Autodesk Fusion 360 part; units mm, degrees
note: some values were not read from the file. Chosen so that the rebuilt part matches the saved one: which bodies a step acts on. Set by a fixed rule: which sketch regions a step uses.
(part 2 of 3)
sketch "Esquisse32" plane through (0, 0, -500) normal (0, 0, -1) x (-1, 0, 0)
  line L0 (-249.6527, -49.4848) -> (-249.7286, -49.4459)
  spline S0 degree 5 poles (-249.7286, -49.4459) (-249.7324, -49.3927) (-249.7363, -49.3397) (-249.7403, -49.2867) (-249.7444, -49.2339) (-249.7485, -49.1812) knots 0.023756 0.023756 0.023756 0.023756 0.023756 0.023756 0.032153 0.032153 0.032153 0.032153 0.032153 0.032153
  spline S1 degree 5 poles (-249.7485, -49.1812) (-249.7705, -49.2534) (-249.7926, -49.3259) (-249.8149, -49.3986) (-249.8372, -49.4715) (-249.8597, -49.5447) knots 0.980595 0.980595 0.980595 0.980595 0.980595 0.980595 0.989283 0.989283 0.989283 0.989283 0.989283 0.989283
  line L1 (-249.8597, -49.5447) -> (-249.8814, -49.5038)
  line L2 (-249.8814, -49.5038) -> (-249.8118, -49.3682)
  spline S2 degree 5 poles (-249.8118, -49.3682) (-249.8339, -49.38) (-249.8559, -49.3918) (-249.878, -49.4036) (-249.9, -49.4154) (-249.922, -49.4272) knots 0 0 0 0 0 0 0.003856 0.003856 0.003856 0.003856 0.003856 0.003856
  spline S3 degree 5 poles (-249.922, -49.4272) (-249.9554, -49.364) (-249.989, -49.3006) (-250.0226, -49.237) (-250.0563, -49.1731) (-250.0901, -49.109) knots 0.991923 0.991923 0.991923 0.991923 0.991923 0.991923 1 1 1 1 1 1
  spline S4 degree 5 poles (-250.0901, -49.109) (-250.1008, -49.1968) (-250.1112, -49.2844) (-250.1213, -49.3717) (-250.1312, -49.4588) (-250.1409, -49.5456) knots 0 0 0 0 0 0 0.013626 0.013626 0.013626 0.013626 0.013626 0.013626
  line L3 (-250.1409, -49.5456) -> (-250.1797, -49.5667)
  spline S5 degree 5 poles (-250.1797, -49.5667) (-251.1535, -48.3219) (-253.072, -45.9257) (-255.5912, -42.9683) (-258.2607, -40.2233) (-260.8003, -38.1712) (-262.454, -37.2128) (-263.5373, -36.7637) (-264.1941, -36.5764) (-264.5063, -36.5108) knots -0.98163 -0.98163 -0.98163 -0.98163 -0.98163 -0.98163 -0.8 -0.6 -0.4 -0.2 0 0 0 0 0 0
  spline S6 degree 5 poles (-264.5063, -36.5108) (-263.9407, -36.3998) (-262.8337, -36.2121) (-261.2449, -36.0334) (-259.2727, -36.0041) (-257.0669, -36.3389) (-255.1423, -37.076) (-253.5194, -38.2446) (-252.2045, -39.8541) (-251.1806, -41.88) (-250.4724, -44.1331) (-250.0804, -46.1405) (-249.8774, -47.72) (-249.7819, -48.7553) (-249.7485, -49.1812) knots -1 -1 -1 -1 -1 -1 -0.9 -0.8 -0.7 -0.6 -0.5 -0.4 -0.3 -0.2 -0.1 -0.032153 -0.032153 -0.032153 -0.032153 -0.032153 -0.032153
  spline S7 degree 5 poles (-249.7485, -49.1812) (-249.2912, -47.6805) (-248.4329, -44.7466) (-247.4586, -40.9967) (-246.7428, -37.2421) (-246.5187, -33.9882) (-246.6822, -32.0838) (-246.9356, -30.9388) (-247.159, -30.2933) (-247.2842, -30) knots -0.980595 -0.980595 -0.980595 -0.980595 -0.980595 -0.980595 -0.8 -0.6 -0.4 -0.2 0 0 0 0 0 0
  spline S8 degree 5 poles (-247.2842, -30) (-246.8689, -30.3996) (-246.0802, -31.1988) (-245.0225, -32.3977) (-243.8673, -33.9965) (-242.8764, -35.9953) (-242.3763, -37.9947) (-242.4027, -39.9944) (-242.9669, -41.9947) (-244.0392, -43.9954) (-245.4301, -45.8049) (-246.7771, -47.2143) (-247.8695, -48.2236) (-248.5742, -48.8326) (-248.821, -49.0413) knots -1 -1 -1 -1 -1 -1 -0.9 -0.8 -0.7 -0.6 -0.5 -0.4 -0.3 -0.2 -0.1 -0.047889 -0.047889 -0.047889 -0.047889 -0.047889 -0.047889
  spline S9 degree 5 poles (-248.821, -49.0413) (-247.5601, -48.3647) (-245.0121, -46.9618) (-241.7841, -45.0562) (-238.692, -42.9485) (-236.2638, -40.8331) (-235.0328, -39.3709) (-234.4024, -38.3821) (-234.1038, -37.7677) (-233.985, -37.4718) knots -0.968205 -0.968205 -0.968205 -0.968205 -0.968205 -0.968205 -0.8 -0.6 -0.4 -0.2 0 0 0 0 0 0
  spline S10 degree 5 poles (-233.985, -37.4718) (-233.9739, -38.0479) (-233.9813, -39.1708) (-234.0812, -40.7664) (-234.3948, -42.7138) (-235.1075, -44.8279) (-236.1676, -46.5953) (-237.6004, -47.9907) (-239.4137, -49.0061) (-241.5866, -49.6626) (-243.9284, -49.9689) (-245.9734, -50.0063) (-247.5642, -49.9319) (-248.6004, -49.8462) (-249.0256, -49.8051) knots -1 -1 -1 -1 -1 -1 -0.9 -0.8 -0.7 -0.6 -0.5 -0.4 -0.3 -0.2 -0.1 -0.032153 -0.032153 -0.032153 -0.032153 -0.032153 -0.032153
  spline S11 degree 5 poles (-249.0256, -49.8051) (-247.6271, -50.5161) (-244.8868, -51.8708) (-241.3631, -53.4815) (-237.7898, -54.8384) (-234.6242, -55.6241) (-232.7204, -55.7938) (-231.5488, -55.743) (-230.8743, -55.6352) (-230.5637, -55.5627) knots -0.980595 -0.980595 -0.980595 -0.980595 -0.980595 -0.980595 -0.8 -0.6 -0.4 -0.2 0 0 0 0 0 0
  spline S12 degree 5 poles (-230.5637, -55.5627) (-231.0293, -55.9023) (-231.9534, -56.5403) (-233.3177, -57.3737) (-235.0928, -58.2338) (-237.2334, -58.8625) (-239.2892, -59.0079) (-241.254, -58.6346) (-243.1259, -57.7316) (-244.91, -56.3282) (-246.5742, -54.509) (-247.8421, -52.746) (-248.755, -51.2735) (-249.3394, -50.243) (-249.6109, -49.7443) knots -1 -1 -1 -1 -1 -1 -0.9 -0.8 -0.7 -0.6 -0.5 -0.4 -0.3 -0.2 -0.1 -0.011578 -0.011578 -0.011578 -0.011578 -0.011578 -0.011578
  spline S13 degree 5 poles (-249.6109, -49.7443) (-249.4929, -49.7574) (-249.3754, -49.7701) (-249.2583, -49.7822) (-249.1417, -49.7939) (-249.0256, -49.8051) knots 0.013626 0.013626 0.013626 0.013626 0.013626 0.013626 0.032153 0.032153 0.032153 0.032153 0.032153 0.032153
  spline S14 degree 5 poles (-249.0256, -49.8051) (-249.1138, -49.7603) (-249.2023, -49.7152) (-249.2913, -49.6698) (-249.3806, -49.6242) (-249.4703, -49.5783) knots 0.980595 0.980595 0.980595 0.980595 0.980595 0.980595 0.99198 0.99198 0.99198 0.99198 0.99198 0.99198
  spline S15 degree 5 poles (-249.4703, -49.5783) (-249.3376, -49.4709) (-249.2064, -49.3635) (-249.0765, -49.2561) (-248.9481, -49.1487) (-248.821, -49.0413) knots 0.021065 0.021065 0.021065 0.021065 0.021065 0.021065 0.047889 0.047889 0.047889 0.047889 0.047889 0.047889
  spline S16 degree 5 poles (-248.821, -49.0413) (-248.9841, -49.1288) (-249.1488, -49.2169) (-249.3152, -49.3056) (-249.4831, -49.3949) (-249.6527, -49.4848) knots 0.968205 0.968205 0.968205 0.968205 0.968205 0.968205 0.989961 0.989961 0.989961 0.989961 0.989961 0.989961
  line L4 (-250.1023, -49.9358) -> (-250.0313, -49.9578)
  spline S17 degree 5 poles (-250.0313, -49.9578) (-250.0413, -49.9451) (-250.0513, -49.9323) (-250.0612, -49.9197) (-250.0712, -49.907) (-250.0812, -49.8943) knots 0 0 0 0 0 0 0.002489 0.002489 0.002489 0.002489 0.002489 0.002489
  line L5 (-250.0812, -49.8943) -> (-250.0337, -49.8013)
  line L6 (-250.0337, -49.8013) -> (-250.0105, -49.7833)
  line L7 (-250.0105, -49.7833) -> (-249.955, -49.8544)
  line L8 (-249.955, -49.8544) -> (-250, -50)
  spline S18 degree 5 poles (-250, -50) (-249.9803, -49.9846) (-249.9606, -49.9691) (-249.941, -49.9537) (-249.9213, -49.9382) (-249.9018, -49.9228) knots 0 0 0 0 0 0 0.003856 0.003856 0.003856 0.003856 0.003856 0.003856
  spline S19 degree 5 poles (-249.9018, -49.9228) (-249.8578, -49.9792) (-249.8138, -50.0358) (-249.7696, -50.0927) (-249.7253, -50.1497) (-249.6809, -50.207) knots 0.991923 0.991923 0.991923 0.991923 0.991923 0.991923 1 1 1 1 1 1
  spline S20 degree 5 poles (-249.6809, -50.207) (-249.6849, -50.1334) (-249.689, -50.06) (-249.6932, -49.9868) (-249.6976, -49.9138) (-249.7021, -49.8411) knots 0 0 0 0 0 0 0.01135 0.01135 0.01135 0.01135 0.01135 0.01135
  spline S21 degree 5 poles (-249.7021, -49.8411) (-248.9612, -51.2322) (-247.49, -53.9208) (-245.5244, -57.2671) (-243.3735, -60.4318) (-241.2297, -62.8927) (-239.7674, -64.1237) (-238.7786, -64.7541) (-238.1643, -65.0527) (-237.8683, -65.1715) knots -0.98124 -0.98124 -0.98124 -0.98124 -0.98124 -0.98124 -0.8 -0.6 -0.4 -0.2 0 0 0 0 0 0
  spline S22 degree 5 poles (-237.8683, -65.1715) (-238.4445, -65.1826) (-239.5673, -65.1752) (-241.163, -65.0753) (-243.1104, -64.7617) (-245.2245, -64.049) (-246.9918, -62.9889) (-248.3872, -61.5561) (-249.4026, -59.7428) (-250.0592, -57.5699) (-250.3654, -55.2281) (-250.4028, -53.1831) (-250.3285, -51.5923) (-250.2427, -50.5561) (-250.2017, -50.1309) knots -1 -1 -1 -1 -1 -1 -0.9 -0.8 -0.7 -0.6 -0.5 -0.4 -0.3 -0.2 -0.1 -0.032153 -0.032153 -0.032153 -0.032153 -0.032153 -0.032153
  spline S23 degree 5 poles (-250.2017, -50.1309) (-250.9126, -51.5294) (-252.2674, -54.2697) (-253.878, -57.7934) (-255.2349, -61.3667) (-256.0206, -64.5323) (-256.1903, -66.4361) (-256.1395, -67.6077) (-256.0317, -68.2822) (-255.9593, -68.5928) knots -0.980595 -0.980595 -0.980595 -0.980595 -0.980595 -0.980595 -0.8 -0.6 -0.4 -0.2 0 0 0 0 0 0
  spline S24 degree 5 poles (-255.9593, -68.5928) (-256.2989, -68.1272) (-256.9369, -67.2031) (-257.7703, -65.8388) (-258.6303, -64.0637) (-259.2591, -61.9231) (-259.3879, -60.1012) (-259.1823, -58.744) (-258.8808, -57.8097) (-258.6501, -57.269) (-258.5758, -57.1069) knots -1 -1 -1 -1 -1 -1 -0.9 -0.8 -0.7 -0.6 -0.5 -0.456879 -0.456879 -0.456879 -0.456879 -0.456879 -0.456879
  spline S25 degree 5 poles (-258.5758, -57.1069) (-258.7531, -57.2839) (-259.561, -58.1021) (-260.775, -59.4308) (-262.0352, -61.0602) (-262.8185, -62.4118) (-263.2676, -63.4951) (-263.4549, -64.1519) (-263.5206, -64.464) knots -0.653826 -0.653826 -0.653826 -0.653826 -0.653826 -0.653826 -0.6 -0.4 -0.2 0 0 0 0 0 0
  spline S26 degree 5 poles (-263.5206, -64.464) (-263.6315, -63.8985) (-263.8192, -62.7915) (-263.998, -61.2027) (-264.0273, -59.2305) (-263.6925, -57.0247) (-262.9554, -55.1001) (-261.7867, -53.4771) (-260.1772, -52.1622) (-258.1513, -51.1384) (-255.8983, -50.4301) (-253.8908, -50.0382) (-252.3113, -49.8352) (-251.276, -49.7397) (-250.8501, -49.7063) knots -1 -1 -1 -1 -1 -1 -0.9 -0.8 -0.7 -0.6 -0.5 -0.4 -0.3 -0.2 -0.1 -0.032153 -0.032153 -0.032153 -0.032153 -0.032153 -0.032153
  spline S27 degree 5 poles (-250.8501, -49.7063) (-252.3508, -49.2489) (-255.2848, -48.3906) (-259.0346, -47.4164) (-262.7892, -46.7005) (-266.029, -46.4775) (-267.9273, -46.6383) (-269.0681, -46.888) (-269.7105, -47.1073) (-270, -47.2287) knots -0.980595 -0.980595 -0.980595 -0.980595 -0.980595 -0.980595 -0.8 -0.6 -0.4 -0.2 -0.004255 -0.004255 -0.004255 -0.004255 -0.004255 -0.004255
  line L9 (-270, -47.2287) -> (-270, -47.2095)
  spline S28 degree 5 poles (-270, -47.2095) (-269.6067, -46.802) (-268.8137, -46.0214) (-267.6211, -44.9712) (-266.0286, -43.822) (-264.036, -42.8342) (-262.0367, -42.334) (-260.0369, -42.3604) (-258.0366, -42.9247) (-256.0359, -43.9969) (-254.0869, -45.4951) (-252.5378, -47.0043) (-251.3889, -48.2878) (-250.6403, -49.1926) (-250.292, -49.6283) knots -0.998432 -0.998432 -0.998432 -0.998432 -0.998432 -0.998432 -0.9 -0.8 -0.7 -0.6 -0.5 -0.4 -0.3 -0.2 -0.1 -0.013022 -0.013022 -0.013022 -0.013022 -0.013022 -0.013022
  spline S29 degree 5 poles (-250.292, -49.6283) (-250.3077, -49.6369) (-250.3234, -49.6456) (-250.3391, -49.6542) (-250.3548, -49.6629) (-250.3704, -49.6715) knots 0.016959 0.016959 0.016959 0.016959 0.016959 0.016959 0.019765 0.019765 0.019765 0.019765 0.019765 0.019765
  spline S30 degree 5 poles (-250.3704, -49.6715) (-250.4671, -49.678) (-250.5634, -49.6846) (-250.6593, -49.6916) (-250.7549, -49.6988) (-250.8501, -49.7063) knots 0.016987 0.016987 0.016987 0.016987 0.016987 0.016987 0.032153 0.032153 0.032153 0.032153 0.032153 0.032153
  spline S31 degree 5 poles (-250.8501, -49.7063) (-250.7965, -49.7226) (-250.7428, -49.739) (-250.6889, -49.7555) (-250.6349, -49.772) (-250.5808, -49.7886) knots 0.980595 0.980595 0.980595 0.980595 0.980595 0.980595 0.987045 0.987045 0.987045 0.987045 0.987045 0.987045
  spline S32 degree 5 poles (-250.5808, -49.7886) (-250.9817, -50.0133) (-251.9101, -50.5515) (-253.2852, -51.4174) (-254.9643, -52.6361) (-256.5642, -54.0996) (-257.6012, -55.3668) (-258.1844, -56.3076) (-258.4778, -56.8931) (-258.5758, -57.1069) knots 0.027348 0.027348 0.027348 0.027348 0.027348 0.027348 0.1 0.2 0.3 0.4 0.456879 0.456879 0.456879 0.456879 0.456879 0.456879
  spline S33 degree 5 poles (-258.5758, -57.1069) (-258.0942, -56.6262) (-256.885, -55.4616) (-255.4179, -54.1468) (-253.6373, -52.6494) (-251.5014, -50.945) (-250.1803, -49.9154) knots 0.653826 0.653826 0.653826 0.653826 0.653826 0.653826 0.8 0.989864 0.989864 0.989864 0.989864 0.989864 0.989864
  spline S34 degree 5 poles (-250.1803, -49.9154) (-250.1847, -49.9586) (-250.189, -50.0018) (-250.1933, -50.0449) (-250.1975, -50.0879) (-250.2017, -50.1309) knots 0.025297 0.025297 0.025297 0.025297 0.025297 0.025297 0.032153 0.032153 0.032153 0.032153 0.032153 0.032153
  spline S35 degree 5 poles (-250.2017, -50.1309) (-250.1819, -50.092) (-250.1621, -50.0531) (-250.1422, -50.0141) (-250.1223, -49.975) (-250.1023, -49.9358) knots 0.980595 0.980595 0.980595 0.980595 0.980595 0.980595 0.985614 0.985614 0.985614 0.985614 0.985614 0.985614
  line L10 (0, 0) -> (-500, 0)
  line L11 (-500, 0) -> (-500, -100)
  line L12 (-500, -100) -> (0, -100)
  line L13 (0, -100) -> (0, 0)
  spline S36 degree 5 poles (-752.6094, 2.3587) (-751.4125, 3.3722) (-749.2008, 5.4108) (-746.6033, 8.4178) (-744.8759, 12.1299) (-745.0448, 16.2519) (-746.2254, 20.0781) (-746.9511, 23.8392) (-746.165, 27.5533) (-743.8381, 30.7762) (-740.6502, 32.8311) (-737.642, 33.0469) (-735.8698, 31.0183) (-736.1134, 26.7853) (-738.8366, 20.7166) (-744.0362, 13.4698) (-751.253, 5.8891) (-759.2111, -0.975) (-766.2809, -6.1031) (-768.9611, -8.1361) (-765.9148, -6.7187) (-760.6181, -3.5743) (-756.3821, -0.6706) (-753.8063, 1.3451) (-752.6094, 2.3587) knots 0 0 0 0 0 0 0.05 0.1 0.15 0.2 0.25 0.3 0.35 0.4 0.45 0.5 0.55 0.6 0.65 0.7 0.75 0.8 0.85 0.9 0.95 1 1 1 1 1 1
  line L14 (-761.998, -2.9349) -> (-767.7728, -7.266)
  spline S37 degree 5 poles (-752.6094, 2.3587) (-752.294, 3.293) (-751.7934, 5.1547) (-751.451, 7.8793) (-751.7283, 11.3123) (-752.6342, 15.4745) (-753.2774, 19.8274) (-752.9808, 24.5534) (-751.5025, 29.4566) (-749.3688, 33.6811) (-747.5009, 36.1011) (-746.8345, 35.7156) (-747.8954, 32.0962) (-750.5345, 25.6604) (-754.1877, 17.3561) (-758.0383, 8.4584) (-761.2107, 0.3317) (-762.9503, -5.7913) (-762.8064, -9.035) (-760.8298, -9.1227) (-757.7438, -6.5899) (-755.2007, -3.2383) (-753.6859, -0.4512) (-752.9248, 1.4243) (-752.6094, 2.3587) knots 0 0 0 0 0 0 0.05 0.1 0.15 0.2 0.25 0.3 0.35 0.4 0.45 0.5 0.55 0.6 0.65 0.7 0.75 0.8 0.85 0.9 0.95 1 1 1 1 1 1
  spline S38 degree 5 poles (-752.6094, 2.3587) (-752.5578, 3.3434) (-752.5781, 5.2711) (-752.9834, 7.9872) (-754.1766, 11.218) (-756.1719, 14.9814) (-757.9657, 18.9993) (-758.9551, 23.6302) (-758.8544, 28.7504) (-757.9396, 33.3939) (-756.794, 36.2281) (-756.0482, 36.0366) (-756.0933, 32.2653) (-756.8982, 25.3561) (-758.1755, 16.3741) (-759.4827, 6.7675) (-760.3449, -1.9137) (-760.368, -8.279) (-759.3543, -11.3636) (-757.4273, -10.9148) (-755.1392, -7.6433) (-753.5946, -3.7299) (-752.8879, -0.6375) (-752.661, 1.3739) (-752.6094, 2.3587) knots 0 0 0 0 0 0 0.05 0.1 0.15 0.2 0.25 0.3 0.35 0.4 0.45 0.5 0.55 0.6 0.65 0.7 0.75 0.8 0.85 0.9 0.95 1 1 1 1 1 1
  spline S39 degree 5 poles (-752.6094, 2.3587) (-752.8254, 3.3208) (-753.365, 5.1716) (-754.4881, 7.6775) (-756.5087, 10.4667) (-759.4454, 13.5522) (-762.2566, 16.9371) (-764.4588, 21.1293) (-765.7433, 26.0868) (-766.1152, 30.8049) (-765.7767, 33.8431) (-765.0069, 33.86) (-764.0328, 30.2163) (-762.9438, 23.3462) (-761.7504, 14.3527) (-760.4173, 4.7496) (-758.9054, -3.8423) (-757.2103, -9.9778) (-755.4019, -12.6745) (-753.6675, -11.7224) (-752.3469, -7.9549) (-751.9154, -3.7699) (-752.0692, -0.6015) (-752.3934, 1.3965) (-752.6094, 2.3587) knots 0 0 0 0 0 0 0.05 0.1 0.15 0.2 0.25 0.3 0.35 0.4 0.45 0.5 0.55 0.6 0.65 0.7 0.75 0.8 0.85 0.9 0.95 1 1 1 1 1 1
  spline S40 degree 5 poles (-752.6094, 2.3587) (-753.0769, 3.2269) (-754.0959, 4.8634) (-755.8534, 6.9734) (-758.5517, 9.114) (-762.2118, 11.2928) (-765.8321, 13.7937) (-769.0836, 17.2363) (-771.658, 21.6634) (-773.289, 26.1062) (-773.7828, 29.1231) (-773.0461, 29.347) (-771.1251, 26.1012) (-768.2229, 19.7797) (-764.6474, 11.4417) (-760.7728, 2.5544) (-756.9989, -5.311) (-753.7114, -10.7617) (-751.2425, -12.8705) (-749.8293, -11.4857) (-749.574, -7.5016) (-750.2876, -3.3554) (-751.2906, -0.346) (-752.1418, 1.4904) (-752.6094, 2.3587) knots 0 0 0 0 0 0 0.05 0.1 0.15 0.2 0.25 0.3 0.35 0.4 0.45 0.5 0.55 0.6 0.65 0.7 0.75 0.8 0.85 0.9 0.95 1 1 1 1 1 1
  spline S41 degree 5 poles (-752.6094, 2.3587) (-753.2938, 3.0685) (-754.7165, 4.3695) (-756.9782, 5.9271) (-760.1539, 7.2603) (-764.2662, 8.3708) (-768.4269, 9.8022) (-772.4867, 12.2399) (-776.16, 15.8083) (-778.9292, 19.6463) (-780.2186, 22.4181) (-779.5697, 22.8325) (-776.8442, 20.2253) (-772.3441, 14.9212) (-766.6515, 7.8571) (-760.5229, 0.3447) (-754.7669, -6.2109) (-750.1307, -10.5724) (-747.1844, -11.9369) (-746.1972, -10.2223) (-747.0263, -6.317) (-748.8321, -2.5171) (-750.6098, 0.1101) (-751.9249, 1.6488) (-752.6094, 2.3587) knots 0 0 0 0 0 0 0.05 0.1 0.15 0.2 0.25 0.3 0.35 0.4 0.45 0.5 0.55 0.6 0.65 0.7 0.75 0.8 0.85 0.9 0.95 1 1 1 1 1 1
  spline S42 degree 5 poles (-752.6094, 2.3587) (-753.46, 2.8576) (-755.1809, 3.7264) (-757.7789, 4.6161) (-761.1965, 5.043) (-765.456, 5.0029) (-769.8486, 5.2587) (-774.4155, 6.5107) (-778.9153, 8.9557) (-782.6174, 11.9042) (-784.6068, 14.2254) (-784.0937, 14.7994) (-780.7658, 13.0243) (-775.0016, 9.131) (-767.6143, 3.8647) (-759.6861, -1.7157) (-752.3748, -6.4752) (-746.7338, -9.4242) (-743.5287, -9.9432) (-743.0407, -8.0257) (-744.8927, -4.489) (-747.6567, -1.3172) (-750.0773, 0.733) (-751.7588, 1.8598) (-752.6094, 2.3587) knots 0 0 0 0 0 0 0.05 0.1 0.15 0.2 0.25 0.3 0.35 0.4 0.45 0.5 0.55 0.6 0.65 0.7 0.75 0.8 0.85 0.9 0.95 1 1 1 1 1 1
  spline S43 degree 5 poles (-752.6094, 2.3587) (-753.5631, 2.6096) (-755.4546, 2.9819) (-758.1963, 3.1376) (-761.6023, 2.6267) (-765.693, 1.4389) (-769.9918, 0.5001) (-774.7271, 0.4735) (-779.7197, 1.6138) (-784.0799, 3.4542) (-786.6218, 5.1525) (-786.2826, 5.8438) (-782.5993, 5.0323) (-775.9984, 2.8385) (-767.4642, -0.2395) (-758.3244, -3.4739) (-750.0002, -6.0843) (-743.7728, -7.402) (-740.5464, -7.037) (-740.5938, -5.0591) (-743.3313, -2.1532) (-746.8486, 0.1553) (-749.7326, 1.4764) (-751.6557, 2.1077) (-752.6094, 2.3587) knots 0 0 0 0 0 0 0.05 0.1 0.15 0.2 0.25 0.3 0.35 0.4 0.45 0.5 0.55 0.6 0.65 0.7 0.75 0.8 0.85 0.9 0.95 1 1 1 1 1 1
  spline S44 degree 5 poles (-752.6094, 2.3587) (-753.5954, 2.343) (-755.5172, 2.1912) (-758.1993, 1.6014) (-761.3412, 0.1905) (-764.9596, -2.0569) (-768.8458, -4.1207) (-773.3983, -5.4239) (-778.5134, -5.6729) (-783.2085, -5.0771) (-786.1143, -4.1275) (-785.9742, -3.3704) (-782.2085, -3.158) (-775.2605, -3.4896) (-766.2123, -4.1509) (-756.5389, -4.7995) (-747.8191, -5.0673) (-741.467, -4.656) (-738.4588, -3.4341) (-739.0381, -1.5422) (-742.4581, 0.5173) (-746.4678, 1.7913) (-749.6013, 2.2853) (-751.6234, 2.3743) (-752.6094, 2.3587) knots 0 0 0 0 0 0 0.05 0.1 0.15 0.2 0.25 0.3 0.35 0.4 0.45 0.5 0.55 0.6 0.65 0.7 0.75 0.8 0.85 0.9 0.95 1 1 1 1 1 1
  spline S45 degree 5 poles (-752.6094, 2.3587) (-753.5546, 2.0775) (-755.3642, 1.4129) (-757.7877, 0.1214) (-760.4324, -2.0849) (-763.3104, -5.2252) (-766.4955, -8.261) (-770.5276, -10.7441) (-775.3859, -12.3639) (-780.0677, -13.0569) (-783.1219, -12.9265) (-783.1912, -12.1597) (-779.6225, -10.9392) (-772.8427, -9.3839) (-763.9517, -7.5795) (-754.4619, -5.5942) (-745.9932, -3.4995) (-739.9877, -1.3897) (-737.4207, 0.5985) (-738.4889, 2.2639) (-742.3378, 3.3244) (-746.5424, 3.4693) (-749.693, 3.0996) (-751.6642, 2.6398) (-752.6094, 2.3587) knots 0 0 0 0 0 0 0.05 0.1 0.15 0.2 0.25 0.3 0.35 0.4 0.45 0.5 0.55 0.6 0.65 0.7 0.75 0.8 0.85 0.9 0.95 1 1 1 1 1 1
  spline S46 degree 5 poles (-752.6094, 2.3587) (-753.4437, 1.8329) (-755.0069, 0.7047) (-756.992, -1.1927) (-758.9434, -4.0308) (-760.8674, -7.8311) (-763.1155, -11.6136) (-766.3281, -15.0925) (-770.5692, -17.9629) (-774.8904, -19.8934) (-777.8665, -20.5919) (-778.1402, -19.8722) (-775.0331, -17.7341) (-768.9243, -14.4073) (-760.8498, -10.2711) (-752.2476, -5.7991) (-744.6581, -1.4972) (-739.4445, 2.1546) (-737.509, 4.7617) (-738.987, 6.0771) (-742.9792, 6.0598) (-747.0671, 5.065) (-750.0011, 3.859) (-751.7751, 2.8844) (-752.6094, 2.3587) knots 0 0 0 0 0 0 0.05 0.1 0.15 0.2 0.25 0.3 0.35 0.4 0.45 0.5 0.55 0.6 0.65 0.7 0.75 0.8 0.85 0.9 0.95 1 1 1 1 1 1
  spline S47 degree 5 poles (-752.6094, 2.3587) (-753.2709, 1.6274) (-754.4717, 0.1192) (-755.8714, -2.2435) (-756.9847, -5.5027) (-757.812, -9.6812) (-758.9562, -13.93) (-761.1111, -18.1466) (-764.4205, -22.0549) (-768.0606, -25.0796) (-770.738, -26.5551) (-771.1956, -25.9359) (-768.7806, -23.0389) (-763.7959, -18.1873) (-757.1367, -12.026) (-750.0601, -5.399) (-743.9126, 0.791) (-739.8776, 5.714) (-738.7173, 8.7466) (-740.4954, 9.6145) (-744.3349, 8.5208) (-748.0027, 6.4599) (-750.5026, 4.507) (-751.9479, 3.09) (-752.6094, 2.3587) knots 0 0 0 0 0 0 0.05 0.1 0.15 0.2 0.25 0.3 0.35 0.4 0.45 0.5 0.55 0.6 0.65 0.7 0.75 0.8 0.85 0.9 0.95 1 1 1 1 1 1
  spline S48 degree 5 poles (-752.6094, 2.3587) (-753.0491, 1.476) (-753.7985, -0.3002) (-754.5088, -2.9529) (-754.7015, -6.3916) (-754.3708, -10.6384) (-754.3262, -15.0383) (-755.2636, -19.68) (-757.3958, -24.3362) (-760.0849, -28.2308) (-762.2649, -30.3739) (-762.8726, -29.9012) (-761.3287, -26.46) (-757.8379, -20.4435) (-753.0879, -12.714) (-748.0616, -4.4235) (-743.8122, 3.1955) (-741.255, 9.0246) (-740.9559, 12.2577) (-742.9022, 12.6137) (-746.3043, 10.5247) (-749.2801, 7.5507) (-751.1603, 4.9958) (-752.1697, 3.2413) (-752.6094, 2.3587) knots 0 0 0 0 0 0 0.05 0.1 0.15 0.2 0.25 0.3 0.35 0.4 0.45 0.5 0.55 0.6 0.65 0.7 0.75 0.8 0.85 0.9 0.95 1 1 1 1 1 1
  spline S49 degree 5 poles (-752.6094, 2.3587) (-752.7946, 1.3901) (-753.037, -0.5224) (-753.0053, -3.2683) (-752.2631, -6.6316) (-750.7989, -10.6317) (-749.5689, -14.8564) (-749.2192, -19.5788) (-750.0162, -24.6376) (-751.5548, -29.1133) (-753.0757, -31.7651) (-753.7884, -31.4739) (-753.2302, -27.7438) (-751.492, -21.0086) (-749.0036, -12.2842) (-746.4005, -2.945) (-744.3642, 5.5379) (-743.4745, 11.8408) (-744.0588, 15.0347) (-746.0289, 14.8524) (-748.7413, 11.923) (-750.8043, 8.2564) (-751.9256, 5.2889) (-752.4241, 3.3272) (-752.6094, 2.3587) knots 0 0 0 0 0 0 0.05 0.1 0.15 0.2 0.25 0.3 0.35 0.4 0.45 0.5 0.55 0.6 0.65 0.7 0.75 0.8 0.85 0.9 0.95 1 1 1 1 1 1
  spline S50 degree 5 poles (-752.6094, 2.3587) (-752.5265, 1.376) (-752.2439, -0.5309) (-751.4725, -3.1665) (-749.8504, -6.2048) (-747.3613, -9.6615) (-745.0371, -13.3977) (-743.4263, -17.8506) (-742.8288, -22.9369) (-743.1028, -27.6617) (-743.8519, -30.6255) (-744.6168, -30.5374) (-745.0856, -26.795) (-745.229, -19.8406) (-745.1867, -10.7684) (-745.1998, -1.0732) (-745.5277, 7.6446) (-746.3715, 13.9537) (-747.7958, 16.8716) (-749.6437, 16.1645) (-751.4651, 12.6119) (-752.4624, 8.5247) (-752.7415, 5.3648) (-752.6923, 3.3413) (-752.6094, 2.3587) knots 0 0 0 0 0 0 0.05 0.1 0.15 0.2 0.25 0.3 0.35 0.4 0.45 0.5 0.55 0.6 0.65 0.7 0.75 0.8 0.85 0.9 0.95 1 1 1 1 1 1
  spline S51 degree 5 poles (-752.6094, 2.3587) (-752.2644, 1.4349) (-751.4778, -0.3252) (-750.024, -2.6549) (-747.6423, -5.1429) (-744.3129, -7.7998) (-741.0669, -10.7704) (-738.3144, -14.6237) (-736.3669, -19.3601) (-735.356, -23.9836) (-735.2776, -27.0396) (-736.0379, -27.1611) (-737.4991, -23.684) (-739.5134, -17.0262) (-741.9204, -8.279) (-744.5487, 1.0532) (-747.2164, 9.3592) (-749.7311, 15.2067) (-751.8899, 17.6321) (-753.4785, 16.4526) (-754.2738, 12.5404) (-754.1315, 8.3357) (-753.5476, 5.2177) (-752.9544, 3.2825) (-752.6094, 2.3587) knots 0 0 0 0 0 0 0.05 0.1 0.15 0.2 0.25 0.3 0.35 0.4 0.45 0.5 0.55 0.6 0.65 0.7 0.75 0.8 0.85 0.9 0.95 1 1 1 1 1 1
  spline S52 degree 5 poles (-752.6094, 2.3587) (-752.028, 1.5622) (-750.7957, 0.0796) (-748.7672, -1.7714) (-745.8026, -3.5246) (-741.8798, -5.1847) (-737.9527, -7.1694) (-734.2628, -10.1372) (-731.1095, -14.1725) (-728.8887, -18.3519) (-727.9888, -21.2734) (-728.6881, -21.5955) (-731.0332, -18.6416) (-734.7691, -12.7741) (-739.4467, -5.0006) (-744.4954, 3.2763) (-749.3051, 10.5546) (-753.3042, 15.5068) (-756.0373, 17.2598) (-757.2488, 15.6955) (-756.9591, 11.7138) (-755.6876, 7.7034) (-754.2842, 4.8585) (-753.1908, 3.1551) (-752.6094, 2.3587) knots 0 0 0 0 0 0 0.05 0.1 0.15 0.2 0.25 0.3 0.35 0.4 0.45 0.5 0.55 0.6 0.65 0.7 0.75 0.8 0.85 0.9 0.95 1 1 1 1 1 1
  spline S53 degree 5 poles (-752.6094, 2.3587) (-751.8346, 1.7486) (-750.2481, 0.6535) (-747.7954, -0.5816) (-744.4678, -1.47) (-740.2425, -2.0102) (-735.9256, -2.8618) (-731.5718, -4.7239) (-727.4468, -7.7589) (-724.1807, -11.1841) (-722.5259, -13.7545) (-723.1124, -14.2534) (-726.1675, -12.0416) (-731.3479, -7.3997) (-737.9493, -1.1765) (-745.0438, 5.4314) (-751.6389, 11.1421) (-756.8258, 14.8318) (-759.9304, 15.7824) (-760.675, 13.9493) (-759.3218, 10.1933) (-757.0154, 6.6747) (-754.8965, 4.314) (-753.3841, 2.9687) (-752.6094, 2.3587) knots 0 0 0 0 0 0 0.05 0.1 0.15 0.2 0.25 0.3 0.35 0.4 0.45 0.5 0.55 0.6 0.65 0.7 0.75 0.8 0.85 0.9 0.95 1 1 1 1 1 1
  spline S54 degree 5 poles (-752.6094, 2.3587) (-751.6988, 1.9802) (-749.8756, 1.3538) (-747.1806, 0.8262) (-743.7367, 0.8686) (-739.5224, 1.4883) (-735.1358, 1.833) (-730.441, 1.2146) (-725.6502, -0.5949) (-721.5811, -3.0119) (-719.2942, -5.0406) (-719.7244, -5.6791) (-723.2629, -4.3737) (-729.5036, -1.3015) (-737.5392, 2.9099) (-746.1534, 7.3587) (-754.0446, 11.0783) (-760.0346, 13.2317) (-763.2806, 13.3094) (-763.503, 11.3434) (-761.1867, 8.0918) (-758.0165, 5.3259) (-755.3393, 3.6244) (-753.52, 2.7371) (-752.6094, 2.3587) knots 0 0 0 0 0 0 0.05 0.1 0.15 0.2 0.25 0.3 0.35 0.4 0.45 0.5 0.55 0.6 0.65 0.7 0.75 0.8 0.85 0.9 0.95 1 1 1 1 1 1
  spline S55 degree 5 poles (-752.6094, 2.3587) (-751.6304, 2.2399) (-749.7059, 2.1286) (-746.9685, 2.3477) (-743.6637, 3.3177) (-739.7729, 5.0514) (-735.642, 6.5668) (-730.9544, 7.238) (-725.853, 6.7881) (-721.2828, 5.5586) (-718.5333, 4.2222) (-718.7752, 3.4912) (-722.5348, 3.7936) (-729.3729, 5.0681) (-738.2468, 6.9553) (-747.7418, 8.915) (-756.3439, 10.3677) (-762.6928, 10.8252) (-765.8394, 10.0243) (-765.5231, 8.0712) (-762.4154, 5.5651) (-758.6165, 3.757) (-755.5795, 2.8409) (-753.5883, 2.4774) (-752.6094, 2.3587) knots 0 0 0 0 0 0 0.05 0.1 0.15 0.2 0.25 0.3 0.35 0.4 0.45 0.5 0.55 0.6 0.65 0.7 0.75 0.8 0.85 0.9 0.95 1 1 1 1 1 1
  spline S56 degree 5 poles (-752.6094, 2.3587) (-751.6347, 2.5085) (-749.7515, 2.9205) (-747.1747, 3.87) (-744.2542, 5.6956) (-740.9754, 8.4148) (-737.4065, 10.9885) (-733.0739, 12.8995) (-728.0403, 13.8426) (-723.3078, 13.8917) (-720.2997, 13.3467) (-720.3355, 12.5775) (-724.0371, 11.8544) (-730.9656, 11.2367) (-740.0195, 10.6598) (-749.6912, 9.9852) (-758.3662, 9.0631) (-764.6031, 7.7907) (-767.417, 6.1706) (-766.5854, 4.3753) (-762.9168, 2.8006) (-758.7711, 2.0845) (-755.5995, 2.0217) (-753.5841, 2.2089) (-752.6094, 2.3587) knots 0 0 0 0 0 0 0.05 0.1 0.15 0.2 0.25 0.3 0.35 0.4 0.45 0.5 0.55 0.6 0.65 0.7 0.75 0.8 0.85 0.9 0.95 1 1 1 1 1 1
  spline S57 degree 5 poles (-752.6094, 2.3587) (-751.7113, 2.7659) (-750.009, 3.6708) (-747.784, 5.2802) (-745.4643, 7.8261) (-743.0408, 11.329) (-740.2986, 14.7702) (-736.6422, 17.7792) (-732.0497, 20.0455) (-727.5059, 21.3695) (-724.4624, 21.6562) (-724.2893, 20.906) (-727.6586, 19.211) (-734.1634, 16.7469) (-742.726, 13.7487) (-751.857, 10.4897) (-759.9616, 7.2613) (-765.6239, 4.3534) (-767.8963, 2.0342) (-766.6112, 0.5298) (-762.6538, 0.0033) (-758.4686, 0.4322) (-755.3977, 1.2275) (-753.5075, 1.9514) (-752.6094, 2.3587) knots 0 0 0 0 0 0 0.05 0.1 0.15 0.2 0.25 0.3 0.35 0.4 0.45 0.5 0.55 0.6 0.65 0.7 0.75 0.8 0.85 0.9 0.95 1 1 1 1 1 1
  spline S58 degree 5 poles (-752.6094, 2.3587) (-751.8544, 2.9931) (-750.4595, 4.3237) (-748.7512, 6.4737) (-747.2044, 9.551) (-745.8158, 13.578) (-744.1037, 17.6314) (-741.3947, 21.5153) (-737.584, 24.9365) (-733.5659, 27.4374) (-730.7126, 28.5346) (-730.3435, 27.8589) (-733.1305, 25.3177) (-738.7294, 21.19) (-746.1655, 15.9928) (-754.0786, 10.3912) (-761.0117, 5.0959) (-765.6795, 0.7682) (-767.2419, -2.0781) (-765.5986, -3.18) (-761.6459, -2.6194) (-757.7316, -1.0771) (-754.9891, 0.5172) (-753.3643, 1.7242) (-752.6094, 2.3587) knots 0 0 0 0 0 0 0.05 0.1 0.15 0.2 0.25 0.3 0.35 0.4 0.45 0.5 0.55 0.6 0.65 0.7 0.75 0.8 0.85 0.9 0.95 1 1 1 1 1 1
  point P0 (-746.5758, 24.0206)
  point P1 (-738.5633, 32.6528)
  point P2 (-764.8854, -5.1005)
  point P3 (-752.6439, 24.8452)
  point P4 (-747.2574, 35.319)
  point P5 (-762.4177, -8.1359)
  point P6 (-758.7094, 24.002)
  point P7 (-756.3485, 35.5407)
  point P8 (-759.2226, -10.393)
  point P9 (-764.3225, 21.5537)
  point P10 (-765.1623, 33.3014)
  point P11 (-755.537, -11.7044)
  point P12 (-769.0669, 17.6817)
  point P13 (-773.045, 28.7673)
  point P14 (-751.6343, -11.9727)
  point P15 (-772.5907, 12.6733)
  point P16 (-779.4122, 22.2745)
  point P17 (-747.8039, -11.1782)
  point P18 (-774.6326, 6.8999)
  point P19 (-783.7915, 14.3047)
  point P20 (-744.3299, -9.3797)
  point P21 (-775.0411, 0.7897)
  point P22 (-785.8582, 5.4488)
  point P23 (-741.4699, -6.7106)
  point P24 (-773.786, -5.2041)
  point P25 (-785.4589, -3.6362)
  point P26 (-739.4362, -3.3689)
  point P27 (-770.9603, -10.6371)
  point P28 (-782.6234, -12.2766)
  point P29 (-738.3794, 0.3975)
  point P30 (-766.7736, -15.1062)
  point P31 (-777.5619, -19.8315)
  point P32 (-738.378, 4.3095)
  point P33 (-761.5364, -18.28)
  point P34 (-770.6497, -25.7408)
  point P35 (-739.432, 8.0767)
  point P36 (-755.6371, -19.9231)
  point P37 (-762.3996, -29.566)
  point P38 (-741.4634, 11.4199)
  point P39 (-749.5133, -19.9137)
  point P40 (-753.4234, -31.0235)
  point P41 (-744.3214, 14.091)
  point P42 (-743.6191, -18.2525)
  point P43 (-744.3868, -30.0052)
  point P44 (-747.7941, 15.892)
  point P45 (-738.3917, -15.0626)
  point P46 (-735.9601, -26.5866)
  point P47 (-751.6239, 16.6893)
  point P48 (-734.2187, -10.5807)
  point P49 (-728.7681, -21.0213)
  point P50 (-755.5269, 16.4238)
  point P51 (-731.4097, -5.1391)
  point P52 (-723.3444, -13.722)
  point P53 (-759.2134, 15.1151)
  point P54 (-730.1729, 0.8585)
  point P55 (-720.0911, -5.2301)
  point P56 (-762.4101, 12.8603)
  point P57 (-730.6002, 6.9675)
  point P58 (-719.2495, 3.8246)
  point P59 (-764.88, 9.8267)
  point P60 (-732.6598, 12.7346)
  point P61 (-720.8821, 12.7707)
  point P62 (-766.4398, 6.2392)
  point P63 (-736.199, 17.7321)
  point P64 (-724.8678, 20.9445)
  point P65 (-766.9739, 2.3638)
  point P66 (-740.9552, 21.5895)
  point P67 (-730.9109, 27.7399)
  point P68 (-766.4426, -1.5118)
  dimension "d135" = 360
  constraint midpoint P2 L14
sketch "Esquisse33" plane through (0, 0, 0) normal (0, 0, 1) x (1, 0, 0)
  line L0 (795, 40) -> (710, 40)
  line L1 (710, 40) -> (710, -35)
  line L2 (710, -35) -> (795, -35)
  line L3 (795, -35) -> (795, 40)
  line L4 (713, -32) -> (792, -32)
  line L5 (792, -32) -> (792, 37)
  line L6 (792, 37) -> (713, 37)
  line L7 (713, 37) -> (713, -32)
  spline S0 degree 5 poles (755, 0) (755.0206, -0.0003) (755.0329, 0.1627) (754.9752, 0.8959) (754.7842, 2.7836) (754.4255, 6.2914) (753.9823, 10.4705) (753.4468, 14.827) (752.7587, 18.9401) (751.7947, 22.5543) (750.4209, 25.5448) (748.5422, 27.882) (746.1587, 29.5972) (743.4086, 30.7504) (740.6479, 31.3947) (738.381, 31.5577) (737.0853, 31.2347) (737.0713, 30.3794) (738.3152, 28.8928) (740.5517, 26.6692) (743.3775, 23.6454) (746.3495, 19.8508) (749.0834, 15.4569) (751.3529, 10.8297) (753.0586, 6.4483) (754.1977, 2.8247) (754.707, 0.9037) (754.9093, 0.1645) (754.9794, 0.0003) (755, 0) knots 0 0 0 0 0 0 0.04 0.08 0.12 0.16 0.2 0.24 0.28 0.32 0.36 0.4 0.44 0.48 0.52 0.56 0.6 0.64 0.68 0.72 0.76 0.8 0.84 0.88 0.92 0.96 1 1 1 1 1 1
  spline S1 degree 5 poles (755, 0) (755.0168, 0.0119) (754.931, 0.151) (754.4533, 0.7102) (753.1892, 2.1251) (750.8372, 4.7522) (748.0223, 7.8727) (745.0284, 11.0824) (742.054, 14.0054) (739.1498, 16.3628) (736.2806, 17.9747) (733.3869, 18.7612) (730.4505, 18.7478) (727.5477, 18.0643) (724.9355, 16.9629) (723.0058, 15.7623) (722.1474, 14.7394) (722.6388, 14.0392) (724.5189, 13.5677) (727.6353, 13.0833) (731.6988, 12.298) (736.3336, 10.975) (741.128, 9.0272) (745.6839, 6.6177) (749.6392, 4.0757) (752.6906, 1.8137) (754.2318, 0.5589) (754.8299, 0.0798) (754.9832, -0.0119) (755, 0) knots 0 0 0 0 0 0 0.04 0.08 0.12 0.16 0.2 0.24 0.28 0.32 0.36 0.4 0.44 0.48 0.52 0.56 0.6 0.64 0.68 0.72 0.76 0.8 0.84 0.88 0.92 0.96 1 1 1 1 1 1
  spline S2 degree 5 poles (755, 0) (755.0067, 0.0195) (754.8554, 0.0816) (754.1403, 0.2532) (752.2859, 0.6549) (748.839, 1.3977) (744.7275, 2.2677) (740.4187, 3.1047) (736.2943, 3.7212) (732.5591, 3.9212) (729.2904, 3.5388) (726.4871, 2.4743) (724.1193, 0.7375) (722.1727, -1.5217) (720.7068, -3.9482) (719.8513, -6.0537) (719.7581, -7.3858) (720.5672, -7.6634) (722.3654, -6.9398) (725.1713, -5.4999) (728.9203, -3.7468) (733.4476, -2.0929) (738.4712, -0.8506) (743.5733, -0.1221) (748.2674, 0.1463) (752.0656, 0.1098) (754.05, 0.0007) (754.8155, -0.0354) (754.9933, -0.0195) (755, 0) knots 0 0 0 0 0 0 0.04 0.08 0.12 0.16 0.2 0.24 0.28 0.32 0.36 0.4 0.44 0.48 0.52 0.56 0.6 0.64 0.68 0.72 0.76 0.8 0.84 0.88 0.92 0.96 1 1 1 1 1 1
  spline S3 degree 5 poles (755, 0) (754.9939, 0.0197) (754.8351, -0.019) (754.1556, -0.3005) (752.4193, -1.0655) (749.194, -2.4906) (745.3564, -4.2034) (741.3786, -6.0589) (737.6795, -7.9844) (734.5401, -10.0181) (732.1204, -12.2488) (730.4782, -14.7577) (729.5835, -17.5546) (729.3366, -20.5265) (729.5769, -23.3512) (730.1224, -25.5574) (730.83, -26.6899) (731.6477, -26.4389) (732.6771, -24.7966) (734.1009, -21.9824) (736.1034, -18.3605) (738.7939, -14.3614) (742.1279, -10.4035) (745.8274, -6.8152) (749.4672, -3.839) (752.5615, -1.6359) (754.231, -0.5579) (754.8716, -0.1371) (755.0061, -0.0197) (755, 0) knots 0 0 0 0 0 0 0.04 0.08 0.12 0.16 0.2 0.24 0.28 0.32 0.36 0.4 0.44 0.48 0.52 0.56 0.6 0.64 0.68 0.72 0.76 0.8 0.84 0.88 0.92 0.96 1 1 1 1 1 1
  spline S4 degree 5 poles (755, 0) (754.9835, 0.0123) (754.8777, -0.1123) (754.4935, -0.7394) (753.5384, -2.3789) (751.7668, -5.4276) (749.6689, -9.069) (747.5414, -12.9082) (745.6806, -16.6403) (744.3361, -20.1309) (743.6897, -23.3577) (743.8358, -26.3528) (744.756, -29.1414) (746.303, -31.6909) (748.1578, -33.8348) (749.8959, -35.2991) (751.134, -35.7994) (751.648, -35.1157) (751.5155, -33.1819) (751.0132, -30.0683) (750.5043, -25.9611) (750.3304, -21.1443) (750.7013, -15.9826) (751.585, -10.9051) (752.7804, -6.3579) (753.9888, -2.7568) (754.7058, -0.9033) (754.9767, -0.1864) (755.0165, -0.0123) (755, 0) knots 0 0 0 0 0 0 0.04 0.08 0.12 0.16 0.2 0.24 0.28 0.32 0.36 0.4 0.44 0.48 0.52 0.56 0.6 0.64 0.68 0.72 0.76 0.8 0.84 0.88 0.92 0.96 1 1 1 1 1 1
  spline S5 degree 5 poles (755, 0) (754.9794, 0.0003) (754.9671, -0.1627) (755.0248, -0.8959) (755.2158, -2.7836) (755.5745, -6.2914) (756.0177, -10.4705) (756.5532, -14.827) (757.2413, -18.9401) (758.2053, -22.5543) (759.5791, -25.5448) (761.4578, -27.882) (763.8413, -29.5972) (766.5914, -30.7504) (769.3521, -31.3947) (771.619, -31.5577) (772.9147, -31.2347) (772.9287, -30.3794) (771.6848, -28.8928) (769.4483, -26.6692) (766.6225, -23.6454) (763.6505, -19.8508) (760.9166, -15.4569) (758.6471, -10.8297) (756.9414, -6.4483) (755.8023, -2.8247) (755.293, -0.9037) (755.0907, -0.1645) (755.0206, -0.0003) (755, 0) knots 0 0 0 0 0 0 0.04 0.08 0.12 0.16 0.2 0.24 0.28 0.32 0.36 0.4 0.44 0.48 0.52 0.56 0.6 0.64 0.68 0.72 0.76 0.8 0.84 0.88 0.92 0.96 1 1 1 1 1 1
  spline S6 degree 5 poles (755, 0) (754.9832, -0.0119) (755.069, -0.151) (755.5467, -0.7102) (756.8108, -2.1251) (759.1628, -4.7522) (761.9777, -7.8727) (764.9716, -11.0824) (767.946, -14.0054) (770.8502, -16.3628) (773.7194, -17.9747) (776.6131, -18.7612) (779.5495, -18.7478) (782.4523, -18.0643) (785.0645, -16.9629) (786.9942, -15.7623) (787.8526, -14.7394) (787.3612, -14.0392) (785.4811, -13.5677) (782.3647, -13.0833) (778.3012, -12.298) (773.6664, -10.975) (768.872, -9.0272) (764.3161, -6.6177) (760.3608, -4.0757) (757.3094, -1.8137) (755.7682, -0.5589) (755.1701, -0.0798) (755.0168, 0.0119) (755, 0) knots 0 0 0 0 0 0 0.04 0.08 0.12 0.16 0.2 0.24 0.28 0.32 0.36 0.4 0.44 0.48 0.52 0.56 0.6 0.64 0.68 0.72 0.76 0.8 0.84 0.88 0.92 0.96 1 1 1 1 1 1
  spline S7 degree 5 poles (755, 0) (754.9933, -0.0195) (755.1446, -0.0816) (755.8597, -0.2532) (757.7141, -0.6549) (761.161, -1.3977) (765.2725, -2.2677) (769.5813, -3.1047) (773.7057, -3.7212) (777.4409, -3.9212) (780.7096, -3.5388) (783.5129, -2.4743) (785.8807, -0.7375) (787.8273, 1.5217) (789.2932, 3.9482) (790.1487, 6.0537) (790.2419, 7.3858) (789.4328, 7.6634) (787.6346, 6.9398) (784.8287, 5.4999) (781.0797, 3.7468) (776.5524, 2.0929) (771.5288, 0.8506) (766.4267, 0.1221) (761.7326, -0.1463) (757.9344, -0.1098) (755.95, -0.0007) (755.1845, 0.0354) (755.0067, 0.0195) (755, 0) knots 0 0 0 0 0 0 0.04 0.08 0.12 0.16 0.2 0.24 0.28 0.32 0.36 0.4 0.44 0.48 0.52 0.56 0.6 0.64 0.68 0.72 0.76 0.8 0.84 0.88 0.92 0.96 1 1 1 1 1 1
  spline S8 degree 5 poles (755, 0) (755.0061, -0.0197) (755.1649, 0.019) (755.8444, 0.3005) (757.5807, 1.0655) (760.806, 2.4906) (764.6436, 4.2034) (768.6214, 6.0589) (772.3205, 7.9844) (775.4599, 10.0181) (777.8796, 12.2488) (779.5218, 14.7577) (780.4165, 17.5546) (780.6634, 20.5265) (780.4231, 23.3512) (779.8776, 25.5574) (779.17, 26.6899) (778.3523, 26.4389) (777.3229, 24.7966) (775.8991, 21.9824) (773.8966, 18.3605) (771.2061, 14.3614) (767.8721, 10.4035) (764.1726, 6.8152) (760.5328, 3.839) (757.4385, 1.6359) (755.769, 0.5579) (755.1284, 0.1371) (754.9939, 0.0197) (755, 0) knots 0 0 0 0 0 0 0.04 0.08 0.12 0.16 0.2 0.24 0.28 0.32 0.36 0.4 0.44 0.48 0.52 0.56 0.6 0.64 0.68 0.72 0.76 0.8 0.84 0.88 0.92 0.96 1 1 1 1 1 1
  spline S9 degree 5 poles (755, 0) (755.0165, -0.0123) (755.1223, 0.1123) (755.5065, 0.7394) (756.4616, 2.3789) (758.2332, 5.4276) (760.3311, 9.069) (762.4586, 12.9082) (764.3194, 16.6403) (765.6639, 20.1309) (766.3103, 23.3577) (766.1642, 26.3528) (765.244, 29.1414) (763.697, 31.6909) (761.8422, 33.8348) (760.1041, 35.2991) (758.866, 35.7994) (758.352, 35.1157) (758.4845, 33.1819) (758.9868, 30.0683) (759.4957, 25.9611) (759.6696, 21.1443) (759.2987, 15.9826) (758.415, 10.9051) (757.2196, 6.3579) (756.0112, 2.7568) (755.2942, 0.9033) (755.0233, 0.1864) (754.9835, 0.0123) (755, 0) knots 0 0 0 0 0 0 0.04 0.08 0.12 0.16 0.2 0.24 0.28 0.32 0.36 0.4 0.44 0.48 0.52 0.56 0.6 0.64 0.68 0.72 0.76 0.8 0.84 0.88 0.92 0.96 1 1 1 1 1 1
  point P0 (753.3997, 14.825)
  point P1 (745, 30)
  point P2 (737.365, 31.0627)
  point P3 (746.2957, 19.6963)
  point P4 (744.9914, 11.053)
  point P5 (729.2763, 18.3927)
  point P6 (722.4748, 14.7646)
  point P7 (736.3809, 10.8184)
  point P8 (740.4061, 3.0592)
  point P9 (723.3781, -0.2401)
  point P10 (720.0081, -7.173)
  point P11 (733.5779, -2.1918)
  point P12 (741.3951, -6.1032)
  point P13 (729.5585, -18.7811)
  point P14 (730.9072, -26.3708)
  point P15 (738.9575, -14.3648)
  point P16 (747.5808, -12.9343)
  point P17 (745.4566, -30.1484)
  point P18 (751.0089, -35.4958)
  point P19 (750.4648, -21.0509)
  point P20 (756.6003, -14.825)
  point P21 (765, -30)
  point P22 (772.635, -31.0627)
  point P23 (763.7043, -19.6963)
  point P24 (765.0086, -11.053)
  point P25 (780.7237, -18.3927)
  point P26 (787.5252, -14.7646)
  point P27 (773.6191, -10.8184)
  point P28 (769.5939, -3.0592)
  point P29 (786.6219, 0.2401)
  point P30 (789.9919, 7.173)
  point P31 (776.4221, 2.1918)
  point P32 (768.6049, 6.1032)
  point P33 (780.4415, 18.7811)
  point P34 (779.0928, 26.3708)
  point P35 (771.0425, 14.3648)
  point P36 (762.4192, 12.9343)
  point P37 (764.5434, 30.1484)
  point P38 (758.9911, 35.4958)
  point P39 (759.5352, 21.0509)
  dimension "d136" = -3
  dimension "d138" = 360
  constraint horizontal L0
  constraint vertical L1
  constraint horizontal L2
  constraint vertical L3
extrude "Extrusion34" add sketch "Esquisse33" along normal blind 10 separate body contours L0 L1 L2 L3 L4 L5 L6 L7 S4 | L4 S3 S4 S5 | S4 S5 S6 | S2 S3 S4 | S5 S6 S7 | S1 S2 S3 | S6 S7 S8 | S0 S1 S2 | S7 S8 S9 | S0 S1 S9 | S0 S8 S9 makes body 15 at (739.3333, 39, 0)
extrude "Extrusion35" add 1 faces at (748.226, -32, 6.6667) along direction (0, -1, 0) blind 3 on bodies 15 bodies 15
extrude "Extrusion36" add 1 faces at (751.3109, -33, 3.3333) along direction (1, 0, 0) blind 0.2 on bodies 15 bodies 15
extrude "Extrusion37" add 1 faces at (751.5109, -34.3535, 3.3333) along direction (1, 0, 0) blind 0.05 on bodies 15 bodies 15
move_body "Déplacer4" bodies 15 to x (1, 0, 0) y (0, 1, 0) z (0, 0, 1) at (-500, 0, 0)
move_body "Déplacer5" bodies 15 to x (1, 0, 0) y (0, 1, 0) z (0, 0, 1) at (0, -100, 500)
sketch "Esquisse34" plane through (0, 0, 1000) normal (0, 0, 1) x (1, 0, 0)
  line L0 (480, -165) -> (20, -165)
  line L1 (20, -165) -> (20, -15)
  line L2 (20, -15) -> (480, -15)
  line L3 (480, -15) -> (480, -165)
  line L4 (500, -185) -> (500, 20)
  line L5 (500, 20) -> (0, 20)
  line L6 (0, 20) -> (0, -185)
  line L7 (0, -185) -> (500, -185)
  line L8 (150, -50) -> (325, -50)
  line L9 (325, -50) -> (325, -125)
  line L10 (325, -125) -> (150, -125)
  line L11 (150, -125) -> (150, -50)
  constraint horizontal L8
  constraint vertical L9
  constraint horizontal L10
  constraint vertical L11
extrude "Extrusion38" add sketch "Esquisse34" against normal blind 20 contours L0 L1 L2 L3 bodies 14
sketch "Esquisse35" plane through (0, 0, 1000) normal (0, 0, 1) x (1, 0, 0)
  line L0 (325, -125) -> (150, -125)
  line L1 (150, -125) -> (150, -50)
  line L2 (150, -50) -> (325, -50)
  line L3 (325, -50) -> (325, -125)
  line L4 (500, -185) -> (500, 20)
  line L5 (500, 20) -> (0, 20)
  line L6 (0, 20) -> (0, -185)
  line L7 (0, -185) -> (500, -185)
  line L8 (155, -50) -> (160, -50)
  line L9 (160, -50) -> (160, -125)
  line L10 (160, -125) -> (155, -125)
  line L11 (155, -125) -> (155, -50)
  line L12 (176.6667, -50) -> (176.6667, -125)
  line L13 (171.6667, -125) -> (171.6667, -50)
  line L14 (171.6667, -50) -> (176.6667, -50)
  line L15 (176.6667, -125) -> (171.6667, -125)
  line L16 (193.3333, -50) -> (193.3333, -125)
  line L17 (188.3333, -125) -> (188.3333, -50)
  line L18 (188.3333, -50) -> (193.3333, -50)
  line L19 (193.3333, -125) -> (188.3333, -125)
  line L20 (210, -50) -> (210, -125)
  line L21 (205, -125) -> (205, -50)
  line L22 (205, -50) -> (210, -50)
  line L23 (210, -125) -> (205, -125)
  line L24 (226.6667, -50) -> (226.6667, -125)
  line L25 (221.6667, -125) -> (221.6667, -50)
  line L26 (221.6667, -50) -> (226.6667, -50)
  line L27 (226.6667, -125) -> (221.6667, -125)
  line L28 (243.3333, -50) -> (243.3333, -125)
  line L29 (238.3333, -125) -> (238.3333, -50)
  line L30 (238.3333, -50) -> (243.3333, -50)
  line L31 (243.3333, -125) -> (238.3333, -125)
  line L32 (260, -50) -> (260, -125)
  line L33 (255, -125) -> (255, -50)
  line L34 (255, -50) -> (260, -50)
  line L35 (260, -125) -> (255, -125)
  line L36 (276.6667, -50) -> (276.6667, -125)
  line L37 (271.6667, -125) -> (271.6667, -50)
  line L38 (271.6667, -50) -> (276.6667, -50)
  line L39 (276.6667, -125) -> (271.6667, -125)
  line L40 (293.3333, -50) -> (293.3333, -125)
  line L41 (288.3333, -125) -> (288.3333, -50)
  line L42 (288.3333, -50) -> (293.3333, -50)
  line L43 (293.3333, -125) -> (288.3333, -125)
  line L44 (310, -50) -> (310, -125)
  line L45 (305, -125) -> (305, -50)
  line L46 (305, -50) -> (310, -50)
  line L47 (310, -125) -> (305, -125)
  line L48 (150, -55) -> (325, -55)
  line L49 (325, -55) -> (325, -60)
  line L50 (325, -60) -> (150, -60)
  line L51 (150, -60) -> (150, -55)
  line L52 (150, -61.6667) -> (325, -61.6667)
  line L53 (325, -61.6667) -> (325, -66.6667)
  line L54 (325, -66.6667) -> (150, -66.6667)
  line L55 (150, -66.6667) -> (150, -61.6667)
  line L56 (150, -68.3333) -> (325, -68.3333)
  line L57 (325, -68.3333) -> (325, -73.3333)
  line L58 (325, -73.3333) -> (150, -73.3333)
  line L59 (150, -73.3333) -> (150, -68.3333)
  line L60 (150, -75) -> (325, -75)
  line L61 (325, -75) -> (325, -80)
  line L62 (325, -80) -> (150, -80)
  line L63 (150, -80) -> (150, -75)
  line L64 (150, -81.6667) -> (325, -81.6667)
  line L65 (325, -81.6667) -> (325, -86.6667)
  line L66 (325, -86.6667) -> (150, -86.6667)
  line L67 (150, -86.6667) -> (150, -81.6667)
  line L68 (150, -88.3333) -> (325, -88.3333)
  line L69 (325, -88.3333) -> (325, -93.3333)
  line L70 (325, -93.3333) -> (150, -93.3333)
  line L71 (150, -93.3333) -> (150, -88.3333)
  line L72 (150, -95) -> (325, -95)
  line L73 (325, -95) -> (325, -100)
  line L74 (325, -100) -> (150, -100)
  line L75 (150, -100) -> (150, -95)
  line L76 (150, -101.6667) -> (325, -101.6667)
  line L77 (325, -101.6667) -> (325, -106.6667)
  line L78 (325, -106.6667) -> (150, -106.6667)
  line L79 (150, -106.6667) -> (150, -101.6667)
  line L80 (150, -108.3333) -> (325, -108.3333)
  line L81 (325, -108.3333) -> (325, -113.3333)
  line L82 (325, -113.3333) -> (150, -113.3333)
  line L83 (150, -113.3333) -> (150, -108.3333)
  line L84 (150, -115) -> (325, -115)
  line L85 (325, -115) -> (325, -120)
  line L86 (325, -120) -> (150, -120)
  line L87 (150, -120) -> (150, -115)
  dimension "d151" = 150
  dimension "d152" = 0
  dimension "d155" = 0
  dimension "d156" = -60
  constraint horizontal L8
  constraint vertical L9
  constraint horizontal L10
  constraint vertical L11
  constraint coincident L0 L9.end
  constraint coincident L2 L8.start
  constraint horizontal L48
  constraint vertical L49
  constraint horizontal L50
  constraint vertical L51
  constraint coincident L3 L49.end
  constraint coincident L1 L48.start
sketch "Esquisse36" plane through (0, 0, 1000) normal (0, 0, 1) x (1, 0, 0)
  line L0 (325, -125) -> (150, -125)
  line L1 (150, -125) -> (150, -50)
  line L2 (150, -50) -> (325, -50)
  line L3 (325, -50) -> (325, -125)
  line L4 (500, -185) -> (500, 20)
  line L5 (500, 20) -> (0, 20)
  line L6 (0, 20) -> (0, -185)
  line L7 (0, -185) -> (500, -185)
  line L8 (150, -60) -> (325, -60)
  line L9 (325, -60) -> (325, -62.5)
  line L10 (325, -62.5) -> (150, -62.5)
  line L11 (150, -62.5) -> (150, -60)
  line L12 (320, -50) -> (317.5, -50)
  line L13 (317.5, -50) -> (317.5, -125)
  line L14 (317.5, -125) -> (320, -125)
  line L15 (320, -125) -> (320, -50)
  dimension "d157" = 2.5
  dimension "d158" = 2.5
  constraint horizontal L8
  constraint vertical L9
  constraint horizontal L10
  constraint vertical L11
  constraint coincident L1 L8.start
  constraint horizontal L12
  constraint vertical L13
  constraint horizontal L14
  constraint vertical L15
  constraint coincident L2 L12.start
  measures "d157" distance of L8.start L10.end
  measures "d158" distance of L12.start L12.end
extrude "Extrusion39" add sketch "Esquisse36" against normal blind 20 separate body contours L3 L8 L9 L10 L15 | L8 L10 L13 L15 | L1 L8 L10 L11 L13 makes body 16
pattern_linear "Réseau R1" count 5 spacing 15 along (0, -1, 0) of bodies 16 makes body 17 at (205.8333, -75, 986.6667) makes body 18 at (205.8333, -90, 986.6667) makes body 19 at (205.8333, -105, 986.6667) makes body 20 at (205.8333, -120, 986.6667)
extrude "Extrusion40" add sketch "Esquisse36" against normal blind 20 separate body contours L0 L10 L13 L14 L15 | L8 L10 L13 L15 | L2 L8 L12 L13 L15 makes body 21
combine "Combiner1" operation add target body 16 tool bodies 17 18 19 20 makes body 22 at (266.6667, -77.5, 993.3333) makes body 23 at (266.6667, -107.5, 993.3333) makes body 24 at (266.6667, -92.5, 993.3333) makes body 25 at (266.6667, -122.5, 993.3333)
pattern_linear "Réseau R2" count 1 spacing 0 along (0, -1, 0) count 7 spacing 26.6667 along (-1, 0, 0) of bodies 21 makes body 26 at (290.8333, -83.3333, 993.3333) makes body 27 at (264.1667, -83.3333, 993.3333) makes body 28 at (237.5, -83.3333, 993.3333) makes body 29 at (210.8333, -83.3333, 993.3333) makes body 30 at (184.1667, -83.3333, 993.3333) makes body 31 at (157.5, -83.3333, 993.3333)
combine "Combiner2" operation add target body 16 tool bodies 21 22 25 28 23 31 30 29 26 24 27
sketch "Esquisse37" plane through (0, 0, 500) normal (0, 0, -1) x (-1, 0, 0)
  line L0 (-100, 240) -> (-500, 240)
  line L1 (-500, 240) -> (-500, -185)
  line L2 (-500, -185) -> (0, -185)
  line L3 (0, -185) -> (0, 20)
  line L4 (0, 20) -> (-100, 20)
  line L5 (-100, 20) -> (-100, 240)
  line L6 (-100, 20) -> (-500, 20)
  constraint coincident L4.end L5.start
  constraint coincident L1 L6.end
  constraint perpendicular L1 L6
sketch "Esquisse38" plane through (500, 0, 0) normal (1, 0, 0) x (0, 0, -1)
  line L0 (-500, 240) -> (-750, 240)
  line L1 (-750, 240) -> (-750, 20)
  line L2 (-750, 20) -> (-1000, 20)
  line L3 (-1000, 20) -> (-1000, -185)
  line L4 (-1000, -185) -> (-500, -185)
  line L5 (-500, -185) -> (-500, 240)
  line L6 (-750, 20) -> (-500, 20)
  constraint coincident L1.end L2.start
  constraint coincident L5 L6.end
  constraint perpendicular L5 L6
split "Scinder4" by plane through (0, 20, 0) normal (0, 1, 0) bodies 14 makes body 32 at (233.3333, 166.6667, 500)
split "Scinder5" by plane through (480, -165, 1000) normal (-1, 0, 0) bodies 14 makes body 33 at (320, -185, 666.6667)
sketch "Esquisse39" plane through (0, -165, 0) normal (0, 1, 0) x (-1, 0, 0)
  line L0 (-20, 980) -> (-480, 980)
  line L1 (-480, 980) -> (-480, 510)
  line L2 (-480, 510) -> (-20, 510)
  line L3 (-20, 510) -> (-20, 980)
  line L4 (-450, 980) -> (-480, 980)
  line L5 (-480, 980) -> (-480, 950)
  line L6 (-480, 950) -> (-450, 950)
  line L7 (-450, 950) -> (-450, 980)
  line L8 (-450, 540) -> (-480, 540)
  line L9 (-480, 540) -> (-480, 510)
  line L10 (-480, 510) -> (-450, 510)
  line L11 (-450, 510) -> (-450, 540)
  constraint horizontal L4
  constraint vertical L5
  constraint horizontal L6
  constraint vertical L7
  constraint coincident L1 L5.end
  constraint coincident L0 L4.start
  constraint horizontal L8
  constraint vertical L9
  constraint horizontal L10
  constraint vertical L11
  constraint coincident L1.end L2.start
extrude "Extrusion41" add sketch "Esquisse39" along normal blind 50 contours L0 L1 L4 L5 L6 L7 | L1 L2 L8 L9 L10 L11 bodies 33